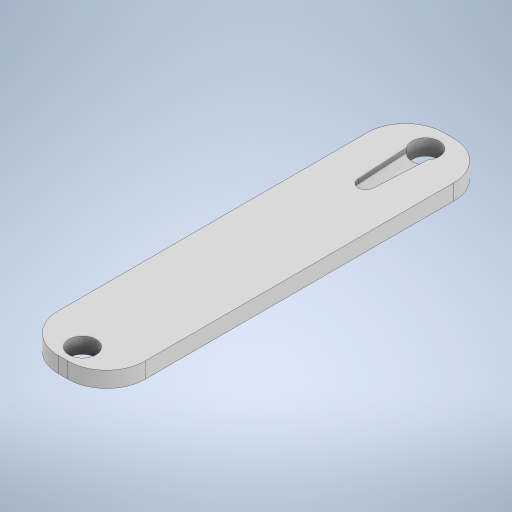
# Autodesk Inventor part: arm_big_part
Saved by Autodesk Inventor 2023 (Build 270158000, 158)
## iProperties
Created: 2023-02-21
Part Number: arm_big_part
Material: Ogólny
Document SubType Name: Modeling
Designer: kamil
Density: 1 g/cm^3
Appearance: Domyślna
Author: kamil
Autodesk Inventor part; units mm, degrees
ref_plane "YZ Plane" through (0, 0, 0) normal (1, 0, 0) x (0, 1, 0)
ref_plane "XZ Plane" through (0, 0, 0) normal (0, 1, 0) x (-1, 0, 0)
ref_plane "XY Plane" through (0, 0, 0) normal (0, 0, 1) x (1, 0, 0)
sketch "Szkic1" plane through (0, 0, 0) normal (0, 1, 0) x (-1, 0, 0)
  line L0 (1.25, 50) -> (-1.25, 50)
  line L1 (-11.25, 40) -> (-11.25, -40)
  line L2 (-1.25, -50) -> (1.25, -50)
  line L3 (11.25, -40) -> (11.25, 40)
  line L4 (11.25, 50) -> (-11.25, -50)
  line L5 (11.25, -50) -> (-11.25, 50)
  arc A0 (11.25, 40) -> (1.25, 50) centre (1.25, 40) ccw
  arc A1 (-1.25, 50) -> (-11.25, 40) centre (-1.25, 40) ccw
  arc A2 (1.25, -50) -> (11.25, -40) centre (1.25, -40) ccw
  arc A3 (-11.25, -40) -> (-1.25, -50) centre (-1.25, -40) ccw
  point P0 (0, 0)
  point P1 (0, 0)
  dimension "d0" = 22.5
  dimension "d1" = 100
  dimension "d2" = 10
  constraints: 12 end point, 8 point on circle, 8 point on line, 8 tangent, 4 centre point, 3 equal radius, 2 parallel, 1 coincident, 1 horizontal, 1 midpoint, 1 perpendicular
  measures "d0" distance of L5.start L4.end
  measures "d1" distance of L4.end L5.end
  measures "d2" radius of A0
extrude "Wyciągnięcie proste1" add sketch "Szkic1" along normal blind 4.1
sketch "Szkic2" plane through (0, 4.1, 0) normal (0, 1, 0) x (1, 0, 0)
  circle A0 centre (0, 44) radius 3.5
  line L0 (1.25, 50) -> (-1.25, 50) projected
  point P0 (0, 0)
  point P1 (0, 50)
  dimension "d5" = 7
  dimension "d14" = 6
  constraints: 1 centre point, 1 midpoint
  measures "d5" diameter of A0
  measures "d14" distance of point (0, 50) A0.centre
extrude "Wyciągnięcie proste2" cut sketch "Szkic2" against normal blind 8
sketch "Szkic3" plane through (0, 4.1, 0) normal (0, 1, 0) x (1, 0, 0)
  line L0 (0, 47.5) -> (0, 28.5)
  arc A0 (-2, 28.5) -> (2, 28.5) centre (0, 28.5) ccw
  line L1 (-2.75, 41.8349) -> (0, 41.8349)
  line L2 (1.25, 50) -> (-1.25, 50) projected
  line L3 (-2, 28.5) -> (-2.75, 41.8349)
  line L4 (2, 28.5) -> (2.75, 41.8349)
  line L5 (0, 41.8349) -> (2.75, 41.8349)
  circle A1 centre (0, 44) radius 3.5 projected
  point P0 (0, 0)
  point P1 (0, 50)
  dimension "d8" = 19
  dimension "d10" = 5.5
  constraints: 10 end point, 4 point on circle, 2 horizontal, 1 centre point, 1 coincident, 1 midpoint, 1 point on line, 1 vertical
  measures "d8" distance of L0.start L0.end
  measures "d10" distance of L1.start L4.end
extrude "Wyciągnięcie proste3" cut sketch "Szkic3" against normal blind 1.1 contours L5 A1 L0 | L0 A1 L1 | A1 L4 A0 L3 picked at (1.6483, 41.6479) picked at (-1.6483, 41.6479)
sketch "Szkic4" plane through (0, 4.1, 0) normal (0, 1, 0) x (1, 0, 0)
  circle A0 centre (0, -45) radius 3.5
  line L0 (-1.25, -50) -> (1.25, -50) projected
  point P0 (0, 0)
  point P1 (0, -50)
  dimension "d15" = 7
  dimension "d16" = 5
  constraints: 1 centre point, 1 midpoint
  measures "d15" diameter of A0
  measures "d16" distance of point (0, -50) A0.centre
extrude "Wyciągnięcie proste4" cut sketch "Szkic4" against normal blind 10
